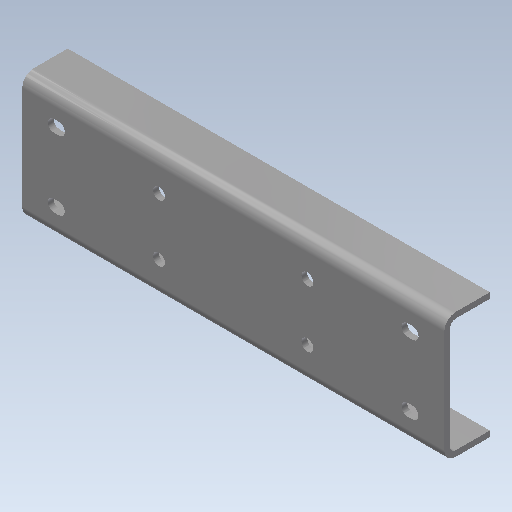
# Autodesk Inventor part: ADSK-MH-10032
Saved by Autodesk Inventor 2020.2 (Build 242310000, 310)
## iProperties
Created: 2008-03-12
Part Number: ADSK-MH-10032
Document SubType Name: Sheet Metal
Designer: R.O'mahony
Density: 7.86 g/cm^3
Mass: 3296.49 g
Surface Area: 1771.73 cm^2
Volume: 419.4 cm^3
Material: Steel, Mild
Sheet Metal Rule: Default
Appearance: Steel
Description: Support Leg Base Plate
Engineer: Demir Ali
Checked By: Demir Ali
Company: Autodesk Ltd
Author: R.O'mahony
Keywords: Roller Conveyor
Revision Number: A
Autodesk Inventor part; units mm, degrees
ref_plane "YZ Plane" through (0, 0, 0) normal (1, 0, 0) x (0, 1, 0)
ref_plane "XZ Plane" through (0, 0, 0) normal (0, 1, 0) x (-1, 0, 0)
ref_plane "XY Plane" through (0, 0, 0) normal (0, 0, 1) x (1, 0, 0)
sketch "Sketch1" plane through (0, 0, 0) normal (0, 0, 1) x (1, 0, 0)
  line L0 (185, -55) -> (-185, -55)
  line L1 (185, 55) -> (-185, 55)
  circle A0 centre (65, -25) radius 5.25
  line L2 (185, 55) -> (185, -55)
  line L3 (-185, 55) -> (-185, -55)
  line L4 (185, 55) -> (-185, -55) construction
  line L5 (185, -55) -> (-185, 55) construction
  line L6 (65, 25) -> (65, -25) construction
  line L7 (152.75, -30.25) -> (157.25, -30.25) construction
  line L8 (152.75, -35.5) -> (157.25, -35.5)
  line L9 (157.25, -25) -> (152.75, -25)
  arc A1 (152.75, -25) -> (152.75, -35.5) centre (152.75, -30.25) ccw
  arc A2 (157.25, -35.5) -> (157.25, -25) centre (157.25, -30.25) ccw
  line L10 (0, 0) -> (155, 0) construction
  line L11 (155, 0) -> (155, -30.25) construction
  dimension "d25" = 50
  dimension "d57" = 2.25
  dimension "d58" = 10.5
  dimension "d59" = 30.25
  dimension "d60" = 155
  dimension "d61" = 110
  dimension "d62" = 370
  dimension "d73" = 65
  constraints: 26 end point, 7 parallel, 5 tangent, 4 point on circle, 3 centre point, 2 midpoint, 1 equal radius, 1 perpendicular, 1 vertical
  measures "d25" distance of L6.end L6.start
  measures "d57" distance of L11.end L7.end
  measures "d58" diameter of A2
  measures "d59" distance of L10.end L11.end
  measures "d60" distance of L10.start L10.end
  measures "d61" distance of L1.start L0.start
  measures "d62" distance of L1.start L1.end
  measures "d73" distance from line of L10.start L6
extrude "Plate1" add sketch "Sketch1" against normal blind 5 contours L0 L3 L1 L2 | A0 | A1 L9 A2 L8
sketch "Sketch4" plane through (185, 50, 0) normal (0, 1, 0) x (-1, 0, 0)
  line L0 (370, 0) -> (0, 0)
  line L1 (0, 0) -> (0, -40)
  line L2 (0, -40) -> (370, -40)
  line L3 (370, -40) -> (370, 0)
  constraints: 4 end point, 4 other
edge flange "Flange1" height 40 angle 90 thickness 5 bend radius 5 thickness toward (0, 1, 0) relief tear relief width 5 relief depth 2.5 corner gap 5 corner form 0 edges at (0, 55, -5) (0, -55, -5) wall of the first edge with corners at (-185, 50, 0) (185, 50, 0) (185, 50, -40) (-185, 50, -40)
bend "Bend3"
corner "Corner3"
extrude "Cut1" cut sketch "Sketch1" against normal blind 5 contours A1 L9 A2 L8
extrude "Cut2" cut sketch "Sketch1" against normal blind 5 contours A0
mirror "Mirror1" about plane through (0, 0, 0) normal (0, 1, 0) of "Cut2", "Cut1"
mirror "Mirror2" about plane through (0, 0, 0) normal (1, 0, 0) of "Cut2", "Cut1", "Mirror1"
equation "\"d74\" = Thickness"
equation "\"d76\" = Thickness"
equation "\"d78\" = Thickness"
equation "\"d63\" = BendReliefWidth"
equation "\"d64\" = BendReliefDepth"
equation "\"d65\" = MinimumRemnant"
equation "\"d66\" = BendRadius"
equation "\"d69\" = BendRadius"
equation "\"d70\" = CornerReliefSize"
equation "\"d71\" = GapSize"
equation "\"d72\" = JacobiRadiusSize"
equation "\"BendRadius\" = Thickness"
equation "\"BendReliefWidth\" = Thickness"
equation "\"BendReliefDepth\" = 0.5 * Thickness"
equation "\"TransitionRadius\" = BendRadius"
equation "\"JacobiRadiusSize\" = Thickness"
equation "\"d36\" = BendRadius"
equation "\"GapSize\" = Thickness"
equation "\"Thickness\" = 5"
equation "\"MinimumRemnant\" = 10"
equation "\"CornerReliefSize\" = 20"
body "Solid1"
